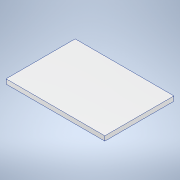
# Autodesk Inventor part: KaretkaYaxis
Saved by Autodesk Inventor 2022 (Build 260153000, 153)
## iProperties
Created: 2023-08-16
Part Number: KaretkaYaxis
Material: Aluminum 6061
Document SubType Name: Modeling
Designer: Kippi
Mass: 1417.5 g
Surface Area: 1142 cm^2
Volume: 525 cm^3
Density: 2.7 g/cm^3
Appearance: Aluminum - Flat
Author: Kippi
Autodesk Inventor part; units mm, degrees
ref_plane "YZ Plane" through (0, 0, 0) normal (1, 0, 0) x (0, 1, 0)
ref_plane "XZ Plane" through (0, 0, 0) normal (0, 1, 0) x (-1, 0, 0)
ref_plane "XY Plane" through (0, 0, 0) normal (0, 0, 1) x (1, 0, 0)
sketch "Sketch1" plane through (0, 0, 0) normal (0, 1, 0) x (-1, 0, 0)
  line L0 (120, 120) -> (-180, 120)
  line L1 (-180, 120) -> (-180, -90)
  line L2 (-180, -90) -> (120, -90)
  line L3 (120, -90) -> (120, 120)
  point P0 (0, 0)
  dimension "d0" = 210
  dimension "d1" = 300
  constraints: 8 end point, 2 parallel, 1 horizontal, 1 perpendicular
  measures "d0" distance of L2.end L0.start
  measures "d1" distance of L1.end L2.end
extrude "Extrusion1" add sketch "Sketch1" along normal blind 14
body "Solid1"
